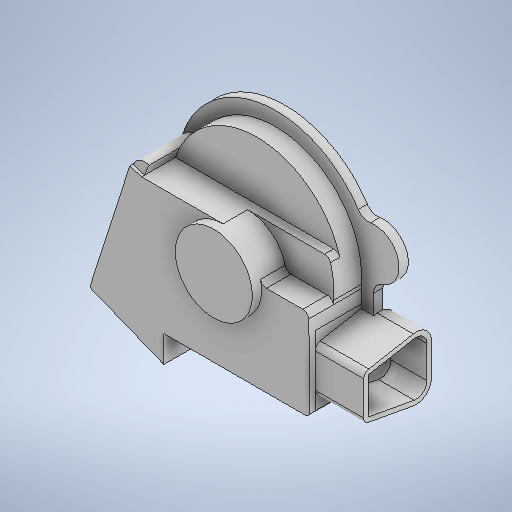
# Autodesk Inventor part: housing susah bf43
Saved by Autodesk Inventor 2025 (Build 290162000, 162)
## iProperties
Created: 2024-09-12
Part Number: housing susah bf43
Material: Generic
Document SubType Name: Modeling
Designer: DMIADX
Density: 1 g/cm^3
Appearance: Default
Author: DMIADX
Autodesk Inventor part; units mm, degrees
ref_plane "YZ Plane" through (0, 0, 0) normal (1, 0, 0) x (0, 1, 0)
ref_plane "XZ Plane" through (0, 0, 0) normal (0, 1, 0) x (-1, 0, 0)
ref_plane "XY Plane" through (0, 0, 0) normal (0, 0, 1) x (1, 0, 0)
sketch "Sketch2" plane through (0, 0, 0) normal (0, 0, 1) x (1, 0, 0)
  line L0 (0, 0) -> (11.764706, 0)
  line L1 (11.764706, 0) -> (11.764706, 22.406178)
  line L2 (11.764706, 22.406178) -> (-0.000086, 22.406178)
  arc A0 (0.44453, 30.876766) -> (-3.538509, 45.934618) centre (0.222222, 38.873676) ccw
  line L3 (-0.000086, 22.406178) -> (-0.000086, 30.41926)
  arc A1 (-7.208869, 43.255825) -> (-6.448611, 43.289555) centre (-6.841013, 43.549313) ccw
  arc A2 (-3.538509, 45.934618) -> (-62.30101, 40.717827) centre (-31.822595, 30.967638) ccw
  line L4 (-75.326836, 0) -> (-62.30101, 40.717827)
  line L5 (0, 0) -> (0, 0)
  line L6 (-5, -5) -> (-18, -5)
  line L7 (-18, -5) -> (-18.975434, -8.640369)
  line L8 (-75.326836, 0) -> (-51.220055, -9.739771)
  line L9 (-75.326836, 0) -> (-49.326836, 0) construction
  line L10 (-51.220055, -9.739771) -> (-24.282436, -12.323433)
  line L11 (-0.000086, 30.876766) -> (0.44453, 30.876766)
  line L12 (-0.000086, 30.876766) -> (-0.000086, 30.41926)
  arc A3 (-24.282436, -12.323433) -> (-18.975434, -8.640369) centre (-23.805063, -7.346274) ccw
  arc A4 (-5, -5) -> (0, 0) centre (-5, 0) ccw
  point P0 (0, -5)
  point P1 (-20.070552, -12.727407)
  dimension "d65" = 5
  constraints: 26 end point, 11 point on circle, 6 tangent, 5 centre point, 5 point on line, 4 perpendicular, 3 horizontal, 2 vertical, 1 equal length, 1 equal radius
  measures "d65" radius of A3
extrude "Extrusion1" add sketch "Sketch2" along normal blind 20
fillet "Fillet1" radius 4 1 edges at (-3.5385, 45.9346, 10)
fillet "Fillet2" radius 4 1 edges at (-0.0001, 30.8768, 10)
fillet_without_effect "Fillet3"
fillet "Fillet4" [suppressed]
fillet "Fillet5" radius 3 1 edges at (-18, -5, 10)
fillet "Fillet6" [suppressed]
fillet "Fillet7" radius 4 1 edges at (-51.2201, -9.7398, 10)
sketch "Sketch3" plane through (0, 0, 20) normal (0, 0, 1) x (1, 0, 0)
  arc A0 (-51.758502, -9.522225) -> (-50.641975, -9.795217) centre (-50.260076, -5.813489) ccw
  line L0 (-50.641975, -9.795217) -> (-24.282436, -12.323433)
  arc A1 (-24.282436, -12.323433) -> (-18.975434, -8.640369) centre (-23.805063, -7.346274) ccw
  line L1 (-18.975434, -8.640369) -> (-18.595797, -7.223543)
  arc A2 (-15.698019, -5) -> (-18.595797, -7.223543) centre (-15.698019, -8) ccw
  line L2 (-15.698019, -5) -> (-5, -5)
  arc A3 (-5, -5) -> (0, 0) centre (-5, 0) ccw
  line L3 (0, 0) -> (11.764706, 0)
  line L4 (11.764706, 0) -> (11.764706, 22.406178)
  line L5 (11.764706, 22.406178) -> (-0.000086, 22.406178)
  line L6 (-0.000086, 22.406178) -> (-0.000086, 27.483811)
  arc A4 (2.740684, 31.280433) -> (-0.000086, 27.483811) centre (3.999914, 27.483811) ccw
  arc A5 (2.740684, 31.280433) -> (-1.074018, 46.767963) centre (0.222222, 38.873676) ccw
  arc A6 (-5.066633, 48.520943) -> (-1.074018, 46.767963) centre (-1.722138, 50.715106) ccw
  arc A7 (-5.066633, 48.520943) -> (-62.30101, 40.717827) centre (-31.822595, 30.967638) ccw
  line L7 (-62.30101, 40.717827) -> (-75.326836, 0)
  line L8 (-75.326836, 0) -> (-51.758502, -9.522225)
  arc A8 (-5.171174, 22.406178) -> (-58.487428, 39.497844) centre (-32.000086, 30.41926) ccw
  line L9 (-0.000086, 22.406178) -> (-5.171174, 22.406178)
  line L10 (-62.30101, 40.717827) -> (-58.487428, 39.497844)
  point P0 (-0.000086, 30.41926)
  dimension "d42" = 56
  constraints: 4 end point, 2 point on circle, 1 centre point, 1 horizontal
  measures "d42" diameter of A8
extrude "Extrusion2" cut sketch "Sketch3" against normal blind 17 contours A7 A6 A5 A4 L6 L9 A8 L10
sketch "Sketch4" plane through (0, 0, 3) normal (0, 0, 1) x (1, 0, 0)
  line L0 (-58.487428, 39.497844) -> (-62.30101, 40.717827)
  circle A0 centre (-58.487428, 39.497844) radius 3.75
  point P0 (0, 0)
  dimension "d45" = 7.5
  constraints: 1 centre point
  measures "d45" diameter of A0
extrude "Extrusion3" add sketch "Sketch4" along normal blind 16
sketch "Sketch5" plane through (0, 0, 20) normal (0, 0, 1) x (1, 0, 0)
  line L0 (-58.487428, 39.497844) -> (-5.512744, 39.497844)
  arc A0 (-5.171174, 22.406178) -> (-57.036726, 42.955873) centre (-32.000086, 30.41926) ccw
  arc A1 (-57.036726, 42.955873) -> (-58.487428, 39.497844) centre (-32.000086, 30.41926) ccw
  arc A2 (-5.512744, 39.497844) -> (-58.487428, 39.497844) centre (-32.000086, 30.41926) ccw
  point P0 (0, 0)
  constraints: 3 point on circle, 2 end point, 1 centre point, 1 concentric, 1 horizontal
extrude "Extrusion4" cut sketch "Sketch5" against normal blind 11
fillet "Fillet8" radius 2 1 edges at (-5.5127, 39.4978, 14.5)
sketch "Sketch6" plane through (0, 0, 3) normal (0, 0, 1) x (1, 0, 0)
  arc A0 (2.740684, 31.280433) -> (-0.000086, 27.483811) centre (3.999914, 27.483811) ccw
  circle A1 centre (-32.000086, 26.997844) radius 12.5
  line L0 (-6.982219, 39.497844) -> (-58.487428, 39.497844)
  point P0 (0, 0)
  dimension "d52" = 25
  constraints: 1 centre point, 1 tangent
  measures "d52" diameter of A1
extrude "Extrusion5" add sketch "Sketch6" along normal blind 20
sketch "Sketch7" plane through (0, 0, 20) normal (0, 0, 1) x (1, 0, 0)
  line L0 (11.764706, 22.406178) -> (-5.171174, 22.406178)
  circle A0 centre (-32.000086, 26.997844) radius 12.5
  line L1 (-19.579675, 28.406178) -> (-4.072546, 28.406178)
  line L2 (-6.982219, 39.497844) -> (-32.000086, 39.497844)
  arc A1 (-5.057768, 38.042351) -> (-6.982219, 39.497844) centre (-6.982219, 37.497844) ccw
  arc A2 (-5.057768, 38.042351) -> (-57.036726, 42.955873) centre (-32.000086, 30.41926) ccw
  arc A3 (-5.057768, 38.042351) -> (-6.982219, 39.497844) centre (-6.982219, 37.497844) ccw
  line L3 (-32.000086, 39.497844) -> (-6.982219, 39.497844)
  arc A4 (-19.579675, 28.406178) -> (-32.000086, 39.497844) centre (-32.000086, 26.997844) ccw
  arc A5 (-5.171174, 22.406178) -> (-5.057768, 38.042351) centre (-32.000086, 30.41926) ccw
  arc A6 (-4.072546, 28.406178) -> (-5.057768, 38.042351) centre (-32.000086, 30.41926) ccw
  point P0 (0, 0)
  point P1 (-11.905746, 28.406178)
  dimension "d55" = 6
  constraints: 7 point on circle, 4 end point, 3 centre point, 2 concentric, 1 horizontal, 1 point on line
  measures "d55" distance from line of L0 point (-11.906, 28.406)
extrude "Extrusion6" cut sketch "Sketch7" against normal blind 8 contours A0 L2 A1 A5 L1
fillet "Fillet9" radius 2 1 edges at (-19.5797, 28.4062, 16)
fillet "Fillet10" radius 5 1 edges at (-5.1712, 22.4062, 11.5)
sketch "Sketch8" plane through (0, 0, 20) normal (0, 0, 1) x (1, 0, 0)
  arc A0 (-5, -5) -> (0, 0) centre (-5, 0) ccw
  line L0 (-15.698019, -5) -> (-5, -5)
  arc A1 (-15.698019, -5) -> (-18.595797, -7.223543) centre (-15.698019, -8) ccw
  line L1 (-18.975434, -8.640369) -> (-18.595797, -7.223543)
  arc A2 (-24.282436, -12.323433) -> (-18.975434, -8.640369) centre (-23.805063, -7.346274) ccw
  line L2 (-50.641975, -9.795217) -> (-24.282436, -12.323433)
  line L3 (-75.326836, 0) -> (-51.758502, -9.522225)
  arc A3 (-51.758502, -9.522225) -> (-50.641975, -9.795217) centre (-50.260076, -5.813489) ccw
  line L4 (-15.698019, -1) -> (-8.467886, -1)
  line L5 (-5, -1) -> (-8.467886, -1)
  arc A4 (-5, -1) -> (-3.85184, 0) centre (-5.091259, 0.263915) ccw
  line L6 (0, 0) -> (11.764706, 0)
  line L7 (-15.698019, -1) -> (-51.210095, -1)
  line L8 (-51.210095, -1) -> (-51.210095, -9.699035)
  line L9 (-51.210095, -9.699035) -> (-24.282436, -12.323433)
  arc A5 (-24.282436, -12.323433) -> (-18.975434, -8.640369) centre (-23.805063, -7.346274) ccw
  arc A6 (-24.282436, -12.323433) -> (-18.975434, -8.640369) centre (-23.805063, -7.346274) ccw
  line L10 (-18.975434, -8.640369) -> (-18.595797, -7.223543)
  arc A7 (-15.698019, -5) -> (-18.595797, -7.223543) centre (-15.698019, -8) ccw
  line L11 (-15.698019, -5) -> (-5, -5)
  arc A8 (-5, -5) -> (0, 0) centre (-5, 0) ccw
  line L12 (-3.85184, 0) -> (0, 0)
  point P0 (-1.464466, -3.535534)
  point P1 (-4.345177, -0.760376)
  dimension "d60" = 4
  dimension "d61" = 4
  constraints: 16 end point, 11 point on circle, 4 centre point, 4 tangent, 3 horizontal, 1 collinear, 1 concentric, 1 parallel
  measures "d60" distance between parallel lines of L0 L4
  measures "d61" distance of point (-1.464, -3.536) point (-4.345, -0.76)
extrude "Extrusion7" cut sketch "Sketch8" against normal blind 17 contours L0 A1 L1 A2 L9 L8 L7 L4 L5 A4 L12 A0
fillet "Fillet11" radius 2 1 edges at (-4.0725, 28.4062, 16)
sketch "Sketch9" plane through (0, 0, 20) normal (0, 0, 1) x (1, 0, 0)
  arc A0 (-5, -1) -> (-3.85184, 0) centre (-5.091259, 0.263915) ccw
  arc A1 (-4.117044, 27.862705) -> (-4.086646, 26.691892) centre (0.862071, 27.406178) ccw
  line L0 (-3.85184, 0) -> (-4.086646, 26.691892)
  line L1 (-0.000086, 22.48107) -> (-0.000086, 27.483811)
  arc A2 (-0.000086, 22.48107) -> (0.862071, 22.406178) centre (0.862071, 27.406178) ccw
  arc A3 (-4.086646, 26.691892) -> (0.862071, 22.406178) centre (0.862071, 27.406178) ccw
  line L2 (11.764706, 22.406178) -> (0.862071, 22.406178)
  line L3 (0.862071, 22.406178) -> (11.764706, 22.406178)
  line L4 (11.764706, 22.406178) -> (11.764706, 0)
  line L5 (11.764706, 0) -> (-3.85184, 0)
  point P0 (0, 0)
  constraints: 8 end point, 2 perpendicular, 2 point on circle, 1 centre point, 1 collinear
extrude "Extrusion8" cut sketch "Sketch9" against normal blind 2
sketch "Sketch10" plane through (0, 0, 0) normal (0, 0, -1) x (-1, 0, 0)
  line L0 (-11.764706, 0) -> (-11.764706, 22.406178)
  line L1 (0, 0) -> (-11.764706, 0)
  line L2 (-11.764706, 0) -> (-11.764706, 22.406178)
  line L3 (-11.764706, 22.406178) -> (0, 22.406178)
  line L4 (0, 22.406178) -> (0, 0)
  constraints: 8 end point, 2 perpendicular, 1 collinear, 1 horizontal
extrude "Extrusion9" add sketch "Sketch10" along normal blind 4
sketch "Sketch11" plane through (11.764706, 0, 18) normal (1, 0, 0) x (0, 0, -1)
  line L0 (0, 11.203089) -> (0, 4.003089)
  line L1 (0, 11.203089) -> (0, 18.403089)
  line L2 (18, 22.406178) -> (22, 22.406178)
  line L3 (0, 18.403089) -> (22, 22.406178)
  line L4 (22, 22.406178) -> (22, 0)
  line L5 (22, 0) -> (0, 4.003089)
  line L6 (0, 4.003089) -> (0, 0)
  line L7 (0, 0) -> (22, 0)
  line L8 (-2, -1) -> (15, -1)
  line L9 (0, 18.403089) -> (0, 22.406178)
  line L10 (0, 22.406178) -> (22, 22.406178)
  point P0 (18, 0)
  dimension "d70" = 7.2
  dimension "d71" = 7.2
  constraints: 18 end point, 2 parallel, 1 perpendicular, 1 vertical
  measures "d70" distance of L0.start L0.end
  measures "d71" distance of L0.start L1.end
extrude "Extrusion10" cut sketch "Sketch11" against normal blind 15.617 contours L5 L7 L6 | L9 L10 L2 L3
fillet "Fillet12" radius 2 2 edges at (3.9562, 4.0031, 18) (3.9562, 18.4031, 18)
fillet "Fillet13" radius 5 2 edges at (5.8824, 0, -4) (5.8824, 22.4062, -4)
sketch "Sketch12" plane through (-3.852294, 0, 0) normal (0, 1, 0) x (1, 0, 0)
  line L0 (3.852294, -3) -> (3.852294, 0)
  line L1 (3.852294, 0) -> (0.020271, 0)
  line L2 (0.020271, 0) -> (0.020271, -3)
  line L3 (3.852294, -3) -> (0.020271, -3)
  constraints: 8 end point, 3 perpendicular
extrude "Extrusion11" add sketch "Sketch12" along normal blind 1.4
sketch "Sketch13" plane through (0, 0, 18) normal (0, 0, 1) x (1, 0, 0)
  line L0 (-3.85184, 0) -> (-4.086646, 26.691892)
  line L1 (0.862071, 22.406178) -> (-3.852294, 22.406178)
  arc A0 (-4.086646, 26.691892) -> (0.862071, 22.406178) centre (0.862071, 27.406178) ccw
  line L2 (0.862071, 22.406178) -> (-4.048945, 22.406178)
  line L3 (-4.086646, 26.691892) -> (-4.048945, 22.406178)
  point P0 (0, 0)
  constraints: 4 end point, 2 point on circle, 2 point on line, 1 centre point, 1 collinear
extrude "Extrusion12" cut sketch "Sketch13" against normal blind 15
sketch "Sketch14" plane through (0, 0, 3) normal (0, 0, 1) x (1, 0, 0)
  line L0 (0.862071, 22.406178) -> (-3.852294, 22.406178)
  arc A0 (-0.000086, 22.48107) -> (0.862071, 22.406178) centre (0.862071, 27.406178) ccw
  line L1 (-0.000086, 22.48107) -> (-0.000086, 22.406178)
  line L2 (-0.000086, 22.406178) -> (0.862071, 22.406178)
  line L3 (-0.000086, 27.483811) -> (-0.000086, 22.48107)
  arc A1 (-0.000086, 22.48107) -> (0.862071, 22.406178) centre (0.862071, 27.406178) ccw
  point P0 (0, 0)
  constraints: 4 end point, 2 point on circle, 1 centre point, 1 collinear, 1 concentric, 1 perpendicular, 1 point on line, 1 tangent
extrude "Extrusion13" cut sketch "Sketch14" against normal blind 30
sketch "Sketch15" plane through (-3.852294, 0, 18) normal (1, 0, 0) x (0, 0, -1)
  arc A0 (1.641962, 18.701858) -> (0, 16.734167) centre (2, 16.734167) ccw
  line L0 (16.104904, 21.333514) -> (1.641962, 18.701858)
  arc A1 (22, 16.414286) -> (16.104904, 21.333514) centre (17, 16.414286) ccw
  line L1 (18, 22.406178) -> (15, 22.406178)
  line L2 (0, 0.051593) -> (0, 22.406178)
  line L3 (18, 22.406178) -> (0, 22.406178)
  line L4 (0, 22.406178) -> (0, 16.734167)
  arc A2 (1.641962, 18.701858) -> (0, 16.734167) centre (2, 16.734167) ccw
  arc A3 (1.641962, 18.701858) -> (0, 16.734167) centre (2, 16.734167) ccw
  line L5 (1.641962, 18.701858) -> (16.104904, 21.333514)
  line L6 (18, 21.313266) -> (18, 22.406178)
  line L7 (15, 22.406178) -> (18, 22.406178)
  line L8 (0, 22.406178) -> (15, 22.406178)
  line L9 (0, 16.734167) -> (0, 22.406178)
  arc A4 (1.641962, 18.701858) -> (0, 16.734167) centre (2, 16.734167) ccw
  line L10 (16.104904, 21.333514) -> (1.641962, 18.701858)
  arc A5 (18, 21.313266) -> (16.104904, 21.333514) centre (17, 16.414286) ccw
  line L11 (18, 22.406178) -> (18, 21.313266)
  line L12 (18, 22.406178) -> (18, 21.313266)
  arc A6 (18, 21.313266) -> (16.104904, 21.333514) centre (17, 16.414286) ccw
  point P0 (18, 0)
  point P1 (18, 21.313266)
  point P2 (18, 22.406178)
  point P3 (15, 22.406178)
  constraints: 10 end point, 4 point on circle, 3 collinear, 3 tangent, 2 centre point, 1 concentric, 1 horizontal, 1 vertical
extrude "Extrusion14" cut sketch "Sketch15" against normal blind 0.197
sketch "Sketch16" plane through (-4.048945, 22.406178, 3) normal (0, -1, 0) x (1, 0, 0)
  line L0 (4.048859, -3) -> (4.048859, 0)
  line L1 (4.048859, -3) -> (-0.000349, -3)
  line L2 (4.048859, -3) -> (4.048859, 0)
  line L3 (4.048859, 0) -> (0, 0)
  line L4 (0, 15) -> (0, 0)
  line L5 (0, 15) -> (-0.000349, 15)
  line L6 (-0.000349, 15) -> (-0.000349, -3)
  line L7 (4.048859, -3) -> (-0.000349, -3)
  line L8 (4.048859, 0) -> (4.048859, -3)
  line L9 (-0.000349, -3) -> (4.048859, -3)
  line L10 (0, 0) -> (-0.000349, -3)
  line L11 (0, 0) -> (4.048859, 0)
  point P0 (4.048945, -3)
  constraints: 8 end point, 2 perpendicular, 1 collinear
sketch "Sketch16 outline for Extrusion15" plane through (-4.048945, 22.406178, 3) normal (0, -1, 0) x (1, 0, 0)
  line L0 (0, 0) -> (-0.000349, -3)
  line L1 (4.048859, 0) -> (0, 0)
  line L2 (4.048859, -3) -> (4.048859, 0)
  line L3 (-0.000349, -3) -> (4.048859, -3)
extrude "Extrusion15" add sketch "Sketch16 outline for Extrusion15" along normal blind 1.4
sketch "Sketch17" plane through (-50.641975, -9.795217, 0) normal (-0.0954746, -0.9954319, 0) x (0.9954319, -0.0954746, 0)
  line L0 (26.480505, 3) -> (-0.574708, 3)
  line L1 (26.480505, 3) -> (26.480505, 20)
  line L2 (0, 20) -> (26.480505, 20)
  line L3 (26.480505, 3) -> (0, 3)
  line L4 (26.480505, 3) -> (26.480505, 20)
  line L5 (0, 20) -> (26.480505, 20)
  line L6 (-0.574708, 3) -> (-0.574708, 20)
  line L7 (0, 0) -> (0, 20)
  line L8 (-0.574708, 20) -> (0, 20)
  point P0 (49.47544, 0)
  constraints: 10 end point, 3 collinear, 1 perpendicular, 1 point on line, 1 vertical
extrude "Extrusion16" cut sketch "Sketch17" against normal blind 1.4
sketch "Sketch18" plane through (11.764706, 5.672011, 18) normal (1, 0, 0) x (0, 0, -1)
  arc A0 (22, 10.742275) -> (16.104904, 15.661503) centre (17, 10.742275) ccw
  line L0 (16.104904, 15.661503) -> (1.641962, 13.029847)
  arc A1 (1.641962, 13.029847) -> (0, 11.062156) centre (2, 11.062156) ccw
  line L1 (0, 11.062156) -> (0, 0)
  arc A2 (0, 0) -> (1.641962, -1.967691) centre (2, 0) ccw
  line L2 (1.641962, -1.967691) -> (16.104904, -4.599348)
  arc A3 (16.104904, -4.599348) -> (22, 0.31988) centre (17, 0.31988) ccw
  line L3 (22, 10.742275) -> (22, 0.31988)
  arc A4 (16.373433, -3.123579) -> (20.5, 0.31988) centre (17, 0.31988) ccw
  line L4 (16.373433, -3.123579) -> (1.91049, -0.491923)
  arc A5 (1.5, 0) -> (1.91049, -0.491923) centre (2, 0) ccw
  line L5 (1.5, 0) -> (1.5, 11.062156)
  arc A6 (1.91049, 11.554078) -> (1.5, 11.062156) centre (2, 11.062156) ccw
  line L6 (1.91049, 11.554078) -> (16.373433, 14.185735)
  arc A7 (20.5, 10.742275) -> (16.373433, 14.185735) centre (17, 10.742275) ccw
  line L7 (20.5, 10.742275) -> (20.5, 0.31988)
  point P0 (18, -5.672011)
  dimension "d88" = 1.5
  constraints: 8 end point, 8 point on circle, 4 centre point, 7 other
  measures "d88" distance between parallel lines of L3 L7
extrude "Extrusion17" cut sketch "Sketch18" against normal blind 11.65 contours L4 A5 L5 A6 L6 A7 L7 A4
body "Solid1"
